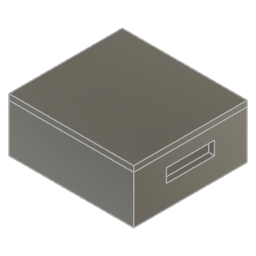
miata-power-switch (Autodesk Fusion 360 design; units mm, degrees)
Autodesk Fusion 360 part; units mm, degrees
sketch "Skizze1" plane through (0, 0, 0) normal (0, 0, 1) x (1, 0, 0) in component "power-switch"
  line L0 (0, 0) -> (65, 0)
  line L1 (65, 0) -> (65, 59)
  line L2 (65, 59) -> (0, 59)
  line L3 (0, 59) -> (0, 0)
  line L4 (32.5, 59) -> (32.5, 0) construction
  line L5 (54.62, 30.875) -> (10.38, 30.875) construction
  line L6 (10.38, 30.875) -> (10.38, 51.125) construction
  line L7 (10.38, 51.125) -> (54.62, 51.125) construction
  line L8 (54.62, 51.125) -> (54.62, 30.875) construction
  line L9 (54.62, 30.875) -> (10.38, 51.125) construction
  line L10 (10.38, 30.875) -> (54.62, 51.125) construction
  line L11 (57.62, 27.875) -> (7.38, 27.875) construction
  line L12 (7.38, 27.875) -> (7.38, 54.125) construction
  line L13 (7.38, 54.125) -> (57.62, 54.125) construction
  line L14 (57.62, 54.125) -> (57.62, 27.875) construction
  line L15 (57.62, 27.875) -> (7.38, 54.125) construction
  line L16 (7.38, 27.875) -> (57.62, 54.125) construction
  line L17 (53.59, 4.45) -> (11.41, 4.45) construction
  line L18 (11.41, 4.45) -> (11.41, 25.55) construction
  line L19 (11.41, 25.55) -> (53.59, 25.55) construction
  line L20 (53.59, 25.55) -> (53.59, 4.45) construction
  line L21 (53.59, 4.45) -> (11.41, 25.55) construction
  line L22 (11.41, 4.45) -> (53.59, 25.55) construction
  line L23 (46.95, 22.84) -> (18.05, 22.84) construction
  line L24 (18.05, 22.84) -> (18.05, 7.16) construction
  line L25 (18.05, 7.16) -> (46.95, 7.16) construction
  line L26 (46.95, 7.16) -> (46.95, 22.84) construction
  line L27 (46.95, 22.84) -> (18.05, 7.16) construction
  line L28 (18.05, 22.84) -> (46.95, 7.16) construction
  circle A0 centre (46.95, 7.16) radius 1
  circle A1 centre (18.05, 22.84) radius 1
  circle A2 centre (10.38, 51.125) radius 1
  circle A3 centre (54.62, 30.875) radius 1
  circle A4 centre (54.62, 51.125) radius 1
  circle A5 centre (10.38, 30.875) radius 1
  line L29 (3, 3) -> (62, 3)
  line L30 (62, 3) -> (62, 56)
  line L31 (62, 56) -> (3, 56)
  line L32 (3, 56) -> (3, 3)
  point P0 (32.5, 41)
  point P1 (32.5, 41)
  point P2 (32.5, 15)
  point P3 (32.5, 15)
  dimension "d56" = 50.24
  dimension "d57" = 26.25
  dimension "d58" = 3
  dimension "d59" = 3
  dimension "d60" = 21.1
  dimension "d61" = 42.18
  dimension "d62" = 6.64
  dimension "d63" = 2.71
  dimension "d64" = 2
  dimension "d65" = 2
  dimension "d66" = 2
  dimension "d67" = 2
  dimension "d68" = 2
  dimension "d69" = 2
  dimension "d70" = 15
  dimension "d71" = 18
  dimension "d72" = 26
  dimension "d73" = 65
  dimension "d74" = -3
  constraint horizontal L0
  constraint vertical L1
  constraint horizontal L2
  constraint vertical L3
  constraint coincident L0.start L3.end
  constraint midpoint L2 L4.start
  constraint midpoint L0 L4.end
  constraint horizontal L5
  constraint perpendicular L5 L6
  constraint parallel L5 L7
  constraint parallel L6 L8
  constraint coincident L9 P1
  constraint coincident L10 P1
  constraint coincident L4 P1
  constraint horizontal L11
  constraint perpendicular L11 L12
  constraint parallel L11 L13
  constraint parallel L12 L14
  constraint coincident L15 P1
  constraint coincident L16 P1
  constraint coincident P1 P0
  constraint horizontal L17
  constraint perpendicular L17 L18
  constraint parallel L17 L19
  constraint parallel L18 L20
  constraint coincident L21 P3
  constraint coincident L22 P3
  constraint coincident L4 P3
  constraint horizontal L23
  constraint perpendicular L23 L24
  constraint parallel L23 L25
  constraint parallel L24 L26
  constraint coincident L27 P3
  constraint coincident L28 P3
  constraint coincident P3 P2
  constraint coincident L25.end L26.start
  constraint coincident L23.end L24.start
  constraint coincident L6.end L7.start
  constraint coincident L5.start L8.end
  constraint coincident L7.end L8.start
  constraint coincident L5.end L6.start
  measures "d56" distance of L12.end L13.end
  measures "d57" distance of L11.start L13.end
  measures "d58" distance of L8 L14
  measures "d59" distance of L7 L13
  measures "d60" distance of L17.start L19.end
  measures "d61" distance of L18.end L19.end
  measures "d62" distance of L20 L26
  measures "d63" distance of L19 L23
  measures "d64" diameter of A0
  measures "d65" diameter of A1
  measures "d66" diameter of A2
  measures "d67" diameter of A3
  measures "d68" diameter of A4
  measures "d69" diameter of A5
  measures "d70" distance of L4.end P3
  measures "d71" distance of L4.start P1
  measures "d72" distance of P1 P3
  measures "d73" distance of L0.start L0.end
extrude "Extrusion1" add sketch "Skizze1" along normal blind 3 contours L29 L30 L31 L32 makes body 1 in component "power-switch"
extrude "Extrusion2" add sketch "Skizze1" along normal blind 25 contours L0 L1 L2 L3 bodies 1 in component "power-switch"
sketch "Skizze2" plane through (0, 0, 25) normal (0, 0, 1) x (-1, 0, 0) in component "power-switch"
  line L0 (-3, -3) -> (-3, -56)
  line L1 (-3, -56) -> (-62, -56)
  line L2 (-62, -56) -> (-62, -3)
  line L3 (-62, -3) -> (-3, -3)
  line L4 (0, -59) -> (0, 0)
  line L5 (0, 0) -> (-65, 0)
  line L6 (-65, 0) -> (-65, -59)
  line L7 (-65, -59) -> (0, -59)
  line L8 (-61, -4) -> (-4, -4)
  line L9 (-4, -4) -> (-4, -55)
  line L10 (-4, -55) -> (-61, -55)
  line L11 (-61, -55) -> (-61, -4)
  dimension "d79" = 1
extrude "Extrusion3" add sketch "Skizze2" along normal blind 4 from surface at -1 separate body contours L8 L9 L10 L11 makes body 2 in component "power-switch"
extrude "Extrusion4" add sketch "Skizze2" along normal blind 3 contours L0 L1 L2 L3 | L4 L5 L6 L7 bodies 2 in component "power-switch"
sketch "Skizze3" plane through (65, 0, 0) normal (1, 0, 0) x (0, 1, 0) in component "power-switch"
  line L0 (0, 0) -> (59, 0)
  line L1 (59, 0) -> (59, 25)
  line L2 (59, 25) -> (0, 25)
  line L3 (0, 25) -> (0, 0)
  line L4 (42, 11.5) -> (17, 11.5)
  line L5 (17, 11.5) -> (17, 18.5)
  line L6 (17, 18.5) -> (42, 18.5)
  line L7 (42, 18.5) -> (42, 11.5)
  line L8 (42, 11.5) -> (17, 18.5) construction
  line L9 (17, 11.5) -> (42, 18.5) construction
  line L10 (0, 15) -> (59, 15) construction
  point P0 (29.5, 15)
  dimension "d85" = 25
  dimension "d86" = 7
  dimension "d87" = 10
  constraint horizontal L4
  constraint perpendicular L4 L5
  constraint parallel L4 L6
  constraint parallel L5 L7
  constraint coincident L8 P0
  constraint coincident L9 P0
  constraint coincident L3 L10.start
  constraint coincident L1 L10.end
  constraint perpendicular L1 L10
  constraint midpoint P0 L10
  measures "d85" distance of L5.end L6.end
  measures "d86" distance of L4.end L5.end
  measures "d87" distance of L1.end L10.end
extrude "Extrusion5" cut sketch "Skizze3" against normal blind 70 contours L4 L5 L6 L7 bodies 1 in component "power-switch"
component "power-switch" placed x (1, 0, 0) y (0, 1, 0) z (0, 0, 1) at (0, 0, 0)
